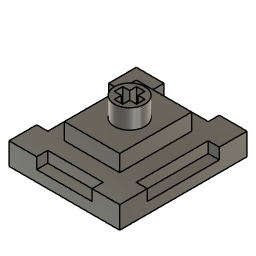
DEL (Autodesk Fusion 360 design; units mm, degrees)
Autodesk Fusion 360 part; units mm, degrees
sketch "スケッチ1" plane through (0, 0, 0) normal (0, 0, 1) x (1, 0, 0)
  line L0 (0, 0) -> (20, 0)
  line L1 (20, 0) -> (20, 23)
  line L2 (20, 23) -> (0, 23)
  line L3 (0, 23) -> (0, 0)
  dimension "d1" = 20
  dimension "d2" = 23
  constraint horizontal L0
  constraint vertical L1
  constraint horizontal L2
  constraint vertical L3
  constraint coincident L0.start L3.end
  measures "d1" distance of L0.start L0.end
  measures "d2" distance of L0.start L2.end
extrude "押し出し1" add sketch "スケッチ1" along normal blind 2
sketch "スケッチ2" plane through (0, 0, 2) normal (0, 0, 1) x (-1, 0, 0)
  line L0 (0, -23) -> (0, 0)
  line L1 (0, 0) -> (-20, 0)
  line L2 (-20, 0) -> (-20, -23)
  line L3 (-20, -23) -> (0, -23)
  line L4 (0, -23) -> (-5, -23)
  line L5 (-5, -23) -> (-5, -18)
  line L6 (-5, -18) -> (0, -18)
  line L7 (0, -18) -> (0, -23)
  line L8 (-20, -23) -> (-15, -23)
  line L9 (-15, -23) -> (-15, -18)
  line L10 (-15, -18) -> (-20, -18)
  line L11 (-20, -18) -> (-20, -23)
  line L12 (0, 0) -> (-5, 0)
  line L13 (-5, 0) -> (-5, -5)
  line L14 (-5, -5) -> (0, -5)
  line L15 (0, -5) -> (0, 0)
  line L16 (-20, 0) -> (-15, 0)
  line L17 (-15, 0) -> (-15, -5)
  line L18 (-15, -5) -> (-20, -5)
  line L19 (-20, -5) -> (-20, 0)
  line L20 (-2, -21) -> (-18, -21)
  line L21 (-18, -21) -> (-18, -2)
  line L22 (-18, -2) -> (-2, -2)
  line L23 (-2, -2) -> (-2, -21)
  dimension "d5" = 5
  dimension "d6" = 5
  dimension "d7" = 5
  dimension "d8" = 5
  dimension "d9" = 5
  dimension "d10" = 5
  dimension "d11" = 5
  dimension "d12" = 5
  constraint horizontal L4
  constraint vertical L5
  constraint horizontal L6
  constraint vertical L7
  constraint coincident L0.start L3.end
  constraint horizontal L8
  constraint vertical L9
  constraint horizontal L10
  constraint vertical L11
  constraint coincident L2.end L3.start
  constraint horizontal L12
  constraint vertical L13
  constraint horizontal L14
  constraint vertical L15
  constraint coincident L0.end L1.start
  constraint horizontal L16
  constraint vertical L17
  constraint horizontal L18
  constraint vertical L19
  constraint coincident L1.end L2.start
  constraint horizontal L20
  constraint vertical L21
  constraint horizontal L22
  constraint vertical L23
  measures "d5" distance of L0.start L4.end
  measures "d6" distance of L0.start L6.end
  measures "d7" distance of L2.end L8.end
  measures "d8" distance of L2.end L10.end
  measures "d9" distance of L0.end L12.end
  measures "d10" distance of L0.end L14.end
  measures "d11" distance of L1.end L16.end
  measures "d12" distance of L1.end L18.end
extrude "押し出し2" add sketch "スケッチ2" along normal blind 2 contours L0 L3 L4 L5 L6 L7 L20 L23 | L0 L1 L12 L13 L14 L15 L22 L23 | L5 L6 L20 L23 | L5 L6 L9 L10 L13 L14 L17 L18 L20 L21 L22 L23 | L2 L3 L8 L9 L10 L11 L20 L21 | L13 L14 L22 L23 | L9 L10 L20 L21 | L1 L2 L16 L17 L18 L19 L21 L22 | L17 L18 L21 L22
sketch "スケッチ3" plane through (0, 0, 4) normal (0, 0, 1) x (-1, 0, 0)
  line L0 (-18, -18) -> (-20, -18)
  line L1 (-20, -18) -> (-20, -23)
  line L2 (-20, -23) -> (-15, -23)
  line L3 (-15, -23) -> (-15, -21)
  line L4 (-15, -21) -> (-5, -21)
  line L5 (-5, -21) -> (-5, -23)
  line L6 (-5, -23) -> (0, -23)
  line L7 (0, -23) -> (0, -18)
  line L8 (0, -18) -> (-2, -18)
  line L9 (-2, -18) -> (-2, -5)
  line L10 (-2, -5) -> (0, -5)
  line L11 (0, -5) -> (0, 0)
  line L12 (0, 0) -> (-5, 0)
  line L13 (-5, 0) -> (-5, -2)
  line L14 (-5, -2) -> (-15, -2)
  line L15 (-15, -2) -> (-15, 0)
  line L16 (-15, 0) -> (-20, 0)
  line L17 (-20, 0) -> (-20, -5)
  line L18 (-20, -5) -> (-18, -5)
  line L19 (-18, -5) -> (-18, -18)
  line L20 (-5, -18) -> (-15, -18)
  line L21 (-15, -18) -> (-15, -5)
  line L22 (-15, -5) -> (-5, -5)
  line L23 (-5, -5) -> (-5, -18)
  constraint horizontal L20
  constraint vertical L21
  constraint horizontal L22
  constraint vertical L23
extrude "押し出し3" add sketch "スケッチ3" along normal blind 3 contours L20 L21 L22 L23
sketch "スケッチ4" plane through (0, 0, 7) normal (0, 0, 1) x (-1, 0, 0)
  line L0 (-5, -5) -> (-15, -5)
  line L1 (-15, -5) -> (-15, -18)
  line L2 (-15, -18) -> (-5, -18)
  line L3 (-5, -18) -> (-5, -5)
  line L4 (-9.55, -13.5) -> (-11.05, -13.5)
  line L5 (-11.05, -13.5) -> (-11.05, -9.5)
  line L6 (-11.05, -9.5) -> (-9.55, -9.5)
  line L7 (-9.55, -9.5) -> (-9.55, -13.5)
  line L8 (-8.3, -12.25) -> (-12.3, -12.25)
  line L9 (-12.3, -12.25) -> (-12.3, -10.75)
  line L10 (-12.3, -10.75) -> (-8.3, -10.75)
  line L11 (-8.3, -10.75) -> (-8.3, -12.25)
  circle A0 centre (-10.3, -11.5) radius 2.75
  dimension "d17" = 13
  dimension "d18" = 1.5
  dimension "d19" = 4
  dimension "d20" = 4
  dimension "d21" = 1.5
  dimension "d22" = 5.5
  constraint horizontal L4
  constraint vertical L5
  constraint horizontal L6
  constraint vertical L7
  constraint horizontal L8
  constraint vertical L9
  constraint horizontal L10
  constraint vertical L11
  measures "d17" distance of L0 L2
  measures "d18" distance of L4.start L4.end
  measures "d19" distance of L4.start L6.end
  measures "d20" distance of L8.start L8.end
  measures "d21" distance of L8.start L10.end
  measures "d22" diameter of A0
extrude "押し出し4" add sketch "スケッチ4" along normal blind 3.5 contours A0
sketch "スケッチ5" plane through (0, 0, 0) normal (0, 0, -1) x (1, 0, 0)
  line L0 (0, 0) -> (0, -23)
  line L1 (0, -23) -> (20, -23)
  line L2 (20, -23) -> (20, 0)
  line L3 (20, 0) -> (0, 0)
  line L4 (16.5, -11.5) -> (13, -15)
  line L5 (13, -8) -> (16.5, -11.5)
  line L6 (13, -15) -> (5, -15)
  line L7 (5, -15) -> (5, -8)
  line L8 (5, -8) -> (13, -8)
  line L9 (7.3948, -12.9209) -> (10.9304, -9.3854)
  line L10 (11.6375, -10.0925) -> (8.102, -13.628)
  line L11 (8.102, -13.628) -> (7.3948, -12.9209)
  line L12 (10.9304, -9.3854) -> (11.6375, -10.0925)
  line L13 (7.3948, -10.0925) -> (8.102, -9.3854)
  line L14 (11.6375, -12.9209) -> (10.9304, -13.628)
  line L15 (10.9304, -13.628) -> (7.3948, -10.0925)
  line L16 (8.102, -9.3854) -> (11.6375, -12.9209)
extrude "押し出し5" cut sketch "スケッチ5" against normal blind 1 contours L4 L5 L6 L7 L8
